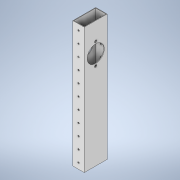
# Autodesk Inventor part: VersaFrame Support for Glock
Saved by Autodesk Inventor 2021 (Build 250183000, 183)
## iProperties
Created: 2020-01-13
Part Number: VersaFrame Support for Glock
Material: Generic
Document SubType Name: Modeling
Designer: aidan
Density: 1 g/cm^3
Appearance: Default
Author: aidan
Autodesk Inventor part; units mm, degrees
ref_plane "YZ Plane" through (0, 0, 0) normal (1, 0, 0) x (0, 1, 0)
ref_plane "XZ Plane" through (0, 0, 0) normal (0, 1, 0) x (-1, 0, 0)
ref_plane "XY Plane" through (0, 0, 0) normal (0, 0, 1) x (1, 0, 0)
sketch "Sketch1" plane through (0, 0, 0) normal (0, 0, 1) x (1, 0, 0)
  line L0 (-12.1708, 16.0073) -> (13.2292, 16.0073)
  line L1 (13.2292, 16.0073) -> (13.2292, -34.7927)
  line L2 (13.2292, -34.7927) -> (-12.1708, -34.7927)
  line L3 (-12.1708, -34.7927) -> (-12.1708, 16.0073)
  line L4 (11.9592, 14.7373) -> (-10.9008, 14.7373)
  line L5 (-10.9008, 14.7373) -> (-10.9008, -33.5227)
  line L6 (-10.9008, -33.5227) -> (11.9592, -33.5227)
  line L7 (11.9592, -33.5227) -> (11.9592, 14.7373)
  point P0 (0, 0)
  dimension "d0" = 25.4
  dimension "d1" = 50.8
  dimension "d2" = 1.27
  constraints: 16 end point, 4 parallel, 2 perpendicular, 1 horizontal, 3 other
  measures "d0" distance of L0.start L0.end
  measures "d1" distance of L0.end L1.end
  measures "d2" distance between parallel lines of L0 L4
extrude "Extrusion1" add sketch "Sketch1" along normal blind 279.4
sketch "Sketch2" plane through (-12.1708, 16.0073, 0) normal (0, 1, 0) x (1, 0, 0)
  circle A0 centre (12.7, -12.7) radius 1.7272
  line L0 (25.4, 0) -> (0, 0) projected
  line L1 (0, 0) -> (0, -279.4) projected
  point P0 (12.1708, 0)
  dimension "d5" = 3.4544
  dimension "d6" = 12.7
  dimension "d7" = 12.7
  constraints: 1 centre point
  measures "d5" diameter of A0
  measures "d6" distance from line of L0 A0.centre
  measures "d7" distance from line of L1 A0.centre
extrude "Extrusion2" cut sketch "Sketch2" against normal through all
pattern_linear "Rectangular Pattern1" count 11 spacing 25.4 along (0, 0, 1) of "Extrusion2"
sketch "Sketch3" plane through (13.2292, -34.7927, 0) normal (1, 0, 0) x (0, 0, -1)
  circle A0 centre (-63.5, 25.4) radius 19.05
  circle A1 centre (-39.6875, 25.4) radius 2.7781
  circle A2 centre (-87.3125, 25.4) radius 2.7781
  circle A3 centre (-63.5, 25.4) radius 23.8125 construction
  line L0 (-63.5, 25.4) -> (0, 25.4) construction
  line L1 (0, 50.8) -> (0, 0) projected
  line L2 (-279.4, 0) -> (-279.4, 50.8) projected
  point P0 (0, 34.7927)
  dimension "d15" = 47.625
  dimension "d16" = 5.5563
  dimension "d17" = 38.1
  dimension "d21" = 215.9
  constraints: 4 centre point, 2 end point, 2 point on circle, 2 point on line, 1 coincident, 1 equal radius, 1 horizontal, 1 midpoint
  measures "d15" diameter of A3
  measures "d16" diameter of A1
  measures "d17" diameter of A0
  measures "d21" distance from line of L2 A0.centre
extrude "Extrusion3" cut sketch "Sketch3" against normal through all
equation "\"d3\" = d13"
equation "\"d13\" = 279.4"
body "Solid1"
